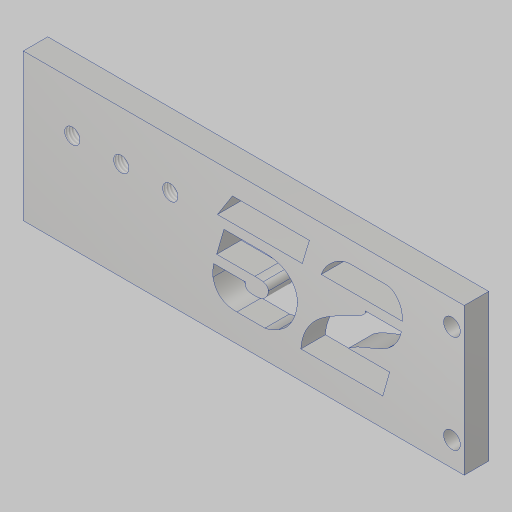
# Autodesk Inventor part: EL2-021
Saved by Autodesk Inventor 2023.5 (Build 275446000, 446)
## iProperties
Created: 2025-01-21
Part Number: EL2-021
Material: Aluminum 6061
Document SubType Name: Modeling
Designer: slick
Density: 2.7 g/cm^3
Appearance: Aluminum - Flat
Author: slick
Autodesk Inventor part; units mm, degrees
ref_plane "YZ Plane" through (0, 0, 0) normal (1, 0, 0) x (0, 1, 0)
ref_plane "XZ Plane" through (0, 0, 0) normal (0, 1, 0) x (-1, 0, 0)
ref_plane "XY Plane" through (0, 0, 0) normal (0, 0, 1) x (1, 0, 0)
sketch "Sketch1" plane through (0, 0, 0) normal (0, 0, 1) x (1, 0, 0)
  line L0 (57.15, -19.05) -> (-57.15, -19.05)
  line L1 (-57.15, -19.05) -> (-57.15, 19.05)
  line L2 (-57.15, 19.05) -> (57.15, 19.05)
  line L3 (57.15, 19.05) -> (57.15, -19.05)
  line L4 (57.15, -19.05) -> (-57.15, 19.05) construction
  line L5 (-57.15, -19.05) -> (57.15, 19.05) construction
  point P0 (0, 0)
  dimension "d0" = 114.3
  dimension "d1" = 38.1
  constraints: 12 end point, 2 midpoint, 2 parallel, 1 horizontal, 1 perpendicular
  measures "d0" distance of L1.end L2.end
  measures "d1" distance of L0.end L1.end
extrude "Extrusion1" add sketch "Sketch1" along normal blind 6.35
sketch "Sketch2" plane through (0, 0, 6.35) normal (0, 0, 1) x (1, 0, 0)
  line L0 (-57.15, 19.05) -> (-57.15, -19.05) projected
  line L1 (57.15, 19.05) -> (-57.15, 19.05) projected
  point P0 (0, 0)
  point P1 (-44.45, 6.35)
  point P2 (-31.75, 6.35)
  point P3 (-19.05, 6.35)
  point P4 (-57.15, 0)
  dimension "d5" = 12.7
  dimension "d6" = 12.7
  dimension "d14" = 12.7
  dimension "d15" = 12.7
  constraints: 2 horizontal alignment, 1 midpoint
  measures "d5" distance of point (-31.75, 6.35) point (-44.45, 6.35)
  measures "d6" distance of point (-31.75, 6.35) point (-19.05, 6.35)
  measures "d14" distance from line of L1 point (-44.45, 6.35)
  measures "d15" distance from line of L0 point (-44.45, 6.35)
hole "Hole1" at (-44.45, 6.35, 6.35) at (-31.75, 6.35, 6.35) at (-19.05, 6.35, 6.35) direction (0, 0, -1) diameter 3.9624 end through all thread size "10-32 UNF" class "2B" standard "ANSI Unified Screw Threads"
sketch "Sketch3" plane through (0, 0, 6.35) normal (0, 0, 1) x (1, 0, 0)
  line L0 (57.15, 19.05) -> (-57.15, 19.05) projected
  line L1 (-57.15, -19.05) -> (57.15, -19.05) projected
  line L2 (57.15, -19.05) -> (57.15, 19.05) projected
  point P0 (0, 0)
  point P1 (53.975, 12.7)
  point P2 (53.975, -12.7)
  dimension "d16" = 6.35
  dimension "d17" = 6.35
  dimension "d18" = 3.175
  constraints: 1 vertical alignment
  measures "d16" distance from line of L0 point (53.975, 12.7)
  measures "d17" distance from line of L1 point (53.975, -12.7)
  measures "d18" distance from line of L2 point (53.975, 12.7)
hole "Hole2" at (53.975, 12.7, 6.35) at (53.975, -12.7, 6.35) direction (0, 0, -1) diameter 4.318 end through all clearance for "Flat Head Machine Screw (82)" size "#8" standard "Ansi Unified Screw Threads"
sketch "Sketch5" plane through (0, 0, 6.35) normal (0, 0, 1) x (1, 0, 0)
  line L0 (-9.5145, 13.6136) -> (35.8392, 13.6136) construction
  line L1 (35.8392, 13.6136) -> (35.8392, -14.7418) construction
  line L2 (35.8392, -14.7418) -> (-9.5145, -14.7418) construction
  line L3 (-9.5145, -14.7418) -> (-9.5145, 13.6136) construction
  spline S0 degree 2 poles (2.8723, -1.5415) (4.408, -1.5415) (5.0344, -1.683) knots 0 0 0 1 1 1
  spline S1 degree 2 poles (5.0344, -1.683) (6.3681, -2.0265) (6.3681, -3.0974) knots 0 0 0 1 1 1
  spline S2 degree 2 poles (6.3681, -3.0974) (6.3681, -4.128) (4.8526, -5.7445) (3.7816, -5.8254) knots 0 0 0 1 2 2 2
  spline S3 degree 2 poles (3.7816, -5.8254) (3.0138, -5.886) (2.5692, -5.886) knots 0 0 0 1 1 1
  spline S4 degree 2 poles (2.5692, -5.886) (0.4273, -5.886) (0.4273, -4.5321) knots 0 0 0 1 1 1
  spline S5 degree 2 poles (0.4273, -4.5321) (0.4273, -4.2694) (0.4677, -4.0067) knots 0 0 0 1 1 1
  line L4 (0.4677, -4.0067) -> (-7.7969, -4.0067)
  spline S6 degree 2 poles (-7.7969, -4.0067) (-8.1606, -6.3305) (-7.9788, -7.159) knots 0 0 0 1 1 1
  spline S7 degree 2 poles (-7.9788, -7.159) (-7.029, -11.8672) (-1.7753, -11.8672) knots 0 0 0 1 1 1
  line L5 (-1.7753, -11.8672) -> (5.479, -11.8672)
  spline S8 degree 2 poles (5.479, -11.8672) (7.1359, -11.6045) (9.0556, -10.3921) knots 0 0 0 1 1 1
  spline S9 degree 2 poles (9.0556, -10.3921) (10.753, -9.3211) (11.5208, -8.331) knots 0 0 0 1 1 1
  spline S10 degree 2 poles (11.5208, -8.331) (13.4405, -5.8456) (13.8446, -2.6731) knots 0 0 0 1 1 1
  spline S11 degree 2 poles (13.8446, -2.6731) (13.885, -2.2488) (13.885, -1.8446) knots 0 0 0 1 1 1
  spline S12 degree 2 poles (13.885, -1.8446) (13.885, 0.3781) (12.713, 1.8128) knots 0 0 0 1 1 1
  spline S13 degree 2 poles (12.713, 1.8128) (11.2986, 3.6516) (7.5805, 5.0257) (4.893, 5.0257) knots 0 0 0 1 2 2 2
  line L6 (4.893, 5.0257) -> (-5.1296, 5.0257)
  line L7 (-5.1296, 5.0257) -> (-7.029, -1.5415)
  line L8 (-7.029, -1.5415) -> (2.8723, -1.5415)
  line L9 (15.1783, 7.4909) -> (-6.827, 7.4909)
  line L10 (-6.827, 7.4909) -> (-2.9271, 13.6136)
  line L11 (-2.9271, 13.6136) -> (17.0171, 13.6136)
  line L12 (17.0171, 13.6136) -> (15.1783, 7.4909)
  line L13 (14.8145, -11.8672) -> (36.0519, -11.8268)
  line L14 (36.0519, -11.8268) -> (37.8301, -5.5627)
  line L15 (37.8301, -5.5627) -> (27.1407, -5.5627)
  spline S14 degree 2 poles (27.1407, -5.5627) (28.6764, -4.2694) (36.0115, -1.4203) (37.527, -0.2887) knots 0 0 0 1 2 2 2
  spline S15 degree 2 poles (37.527, -0.2887) (40.1539, 1.7724) (40.841, 5.0257) knots 0 0 0 1 1 1
  line L16 (40.841, 5.0257) -> (31.5256, 5.0257)
  spline S16 degree 2 poles (31.5256, 5.0257) (31.566, 4.9449) (31.566, 4.8438) knots 0 0 0 1 1 1
  spline S17 degree 2 poles (31.566, 4.8438) (31.566, 3.8133) (27.7267, 1.9947) knots 0 0 0 1 1 1
  spline S18 degree 2 poles (27.7267, 1.9947) (22.0486, -0.6524) (19.7248, -2.6125) knots 0 0 0 1 1 1
  spline S19 degree 2 poles (19.7248, -2.6125) (15.1783, -6.3709) (14.8145, -11.8672) knots 0 0 0 1 1 1
  spline S20 degree 2 poles (41.1441, 7.4909) (41.1441, 9.7743) (40.4166, 11.0676) knots 0 0 0 1 1 1
  spline S21 degree 2 poles (40.4166, 11.0676) (39.0021, 13.6136) (36.9006, 13.6136) knots 0 0 0 1 1 1
  line L17 (36.9006, 13.6136) -> (27.8682, 13.6136)
  spline S22 degree 2 poles (27.8682, 13.6136) (25.4433, 13.6136) (20.8968, 9.8956) (20.0885, 7.4909) knots 0 0 0 1 2 2 2
  line L18 (20.0885, 7.4909) -> (41.1441, 7.4909)
  point P0 (0, 0)
  constraints: 2 other
emboss "Emboss2" sketch "Sketch5" operation cut depth 6.35 direction (0, 0, -1)
equation "\"d5\" = d4"
equation "\"d6\" = d4"
equation "\"d4\" = 12.7"
body "Solid1"
